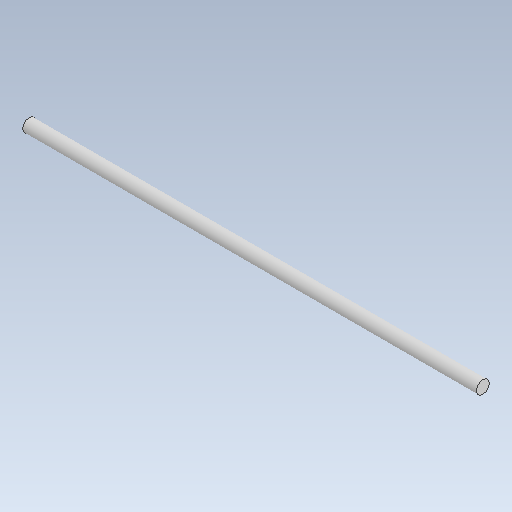
# Autodesk Inventor part: axle_example
Saved by Autodesk Inventor 2021 (Build 250183000, 183)
## iProperties
Created: 2021-06-02
Part Number: axle_example
Material: Generic
Document SubType Name: Modeling
Density: 1 g/cm^3
Appearance: Default
Autodesk Inventor part; units mm, degrees
ref_plane "YZ Plane" through (0, 0, 0) normal (1, 0, 0) x (0, 1, 0)
ref_plane "XZ Plane" through (0, 0, 0) normal (0, 1, 0) x (-1, 0, 0)
ref_plane "XY Plane" through (0, 0, 0) normal (0, 0, 1) x (1, 0, 0)
sketch "Sketch1" plane through (0, 0, 0) normal (1, 0, 0) x (0, 1, 0)
  circle A0 centre (0, 0) radius 9
  dimension "d0" = 18
  constraints: 1 centre point, 1 coincident
  measures "d0" diameter of A0
extrude "Extrusion1" add sketch "Sketch1" along normal mid plane 635
equation "\"d0\" = 2 * secure_arm_radii"
equation "\"d1\" = wheelchair_deployed_width"
equation "\"hoop_angle_z\" = 45deg"
equation "\"hoop_bearing_length\" = 5deg"
equation "\"hoop_cable_diam\" = 5"
equation "\"hoop_cable_pulley_diam\" = 22"
equation "\"hoop_thickness_large\" = 4"
equation "\"hoop_thickness_medium\" = 3.2"
equation "\"hoop_thickness_small\" = 2"
equation "\"hoop_width_large\" = 51"
equation "\"hoop_width_medium\" = 33.7"
equation "\"hoop_width_small\" = 25.4"
equation "\"rack_tooth_addendum\" = 5"
equation "\"rack_tooth_dedendum\" = 5"
equation "\"rack_tooth_thickness\" = 5"
equation "\"secure_arm_angle\" = 35deg"
equation "\"secure_arm_radii\" = 9"
equation "\"support_baseClamp_platformLengthBuffer\" = 35"
equation "\"support_baseClamp_platformThickness\" = 15"
equation "\"support_baseClamp_platformWidthBuffer\" = 0"
equation "\"support_baseClamp_sleeveHoleDiameter\" = 12"
equation "\"support_baseClamp_sleeveSweepTerminationAngle\" = 55deg"
equation "\"support_baseClamp_thickness\" = 8"
equation "\"support_frame_endHoleBuffer\" = 45"
equation "\"support_frame_squareBarFillet\" = 2"
equation "\"support_frame_squareBarThickness\" = 5"
equation "\"hoop_tabs_thickness\" = 6"
equation "\"hoop_tabs_hole\" = 12"
equation "\"wheelchair_deployed_width\" = 635"
equation "\"wheelchair_deployed_length\" = 1067"
equation "\"wheelchair_deployed_height\" = 914"
equation "\"sm_varx_squareBarThickness\" = 2.5"
equation "\"sm_varx_pinPlate_thickness\" = 5"
equation "\"sm_varx_pinPlate_holeDiameter\" = 5"
equation "\"sm_varx_member_tolerance\" = 0.5"
equation "\"hoop_bushing23_radialInterference\" = 0"
equation "\"hoop_bushing12_radialInterference\" = 0"
equation "\"hoop_bushing12_od\" = -2 * hoop_thickness_large + hoop_width_large + hoop_bushing12_radialInterference"
equation "\"hoop_bushing23_od\" = -2 * hoop_thickness_medium + hoop_width_medium + hoop_bushing23_radialInterference"
equation "\"wheelchatir_pos_deploy_angle_0\" = 65deg"
equation "\"wheelchatir_pos_store_angle_0\" = 90deg"
equation "\"wheelchatir_pos_deploy_angle_1\" = 20deg"
equation "\"wheelchatir_pos_store_angle_1\" = 20deg"
equation "\"hoop_bushing12_thickness\" = -hoop_width_medium + hoop_bushing12_od - 2 * hoop_bushing12_radialInterference"
equation "\"hoop_bushing23_thickness\" = -hoop_width_small + hoop_bushing23_od - 2 * hoop_bushing23_radialInterference"
body "Solid1"
